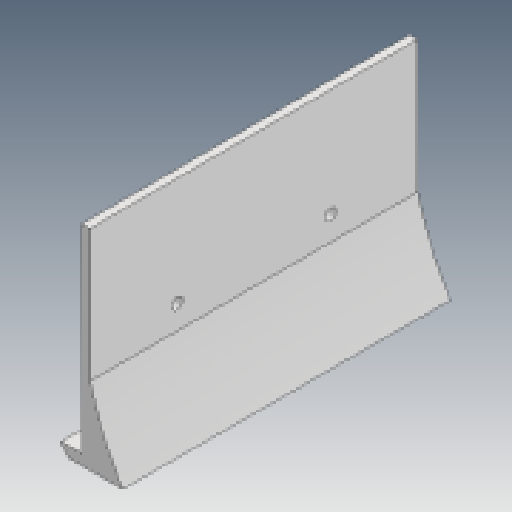
# Autodesk Inventor part: Rampa
Saved by Autodesk Inventor 2026.1 (Build 301233020, 233B)
## iProperties
Created: 2025-11-13
Part Number: Rampa
Material: Genérico
Document SubType Name: Modeling
Designer: Emmanuel Ribeiro
Density: 1 g/cm^3
Appearance: Padrão
Author: Emmanuel Ribeiro
Autodesk Inventor part; units mm, degrees
ref_plane "YZ Plane" through (0, 0, 0) normal (1, 0, 0) x (0, 1, 0)
ref_plane "XZ Plane" through (0, 0, 0) normal (0, 1, 0) x (-1, 0, 0)
ref_plane "XY Plane" through (0, 0, 0) normal (0, 0, 1) x (1, 0, 0)
sketch "Esboço1" plane through (0, 0, 0) normal (0, 0, 1) x (1, 0, 0)
  line L0 (0, 0) -> (10, 0)
  line L1 (0, 51.1555) -> (0, 0)
  line L2 (2, 35) -> (2, 18.8445)
  line L3 (2, 35) -> (2, 51.1555)
  arc A0 (2, 18.8445) -> (10, 0) centre (66.25, 35) ccw
  line L4 (2, 51.1555) -> (0, 51.1555)
  constraints: 10 end point, 2 perpendicular, 2 point on circle, 1 centre point, 1 horizontal
extrude "Extrusão1" add sketch "Esboço1" along normal blind 80
sketch "Esboço2" plane through (0, 0, 80) normal (0, 0, 1) x (1, 0, 0)
  line L0 (0, 0) -> (10, 0) projected
  line L1 (0, 0) -> (-3, 0)
  line L2 (-5, 2) -> (-5, 2.6)
  line L3 (-5, 2.6) -> (0, 2.6)
  line L4 (-3, 0) -> (-5, 2)
  line L5 (0, 51.1555) -> (0, 0) projected
  line L6 (0, 2.6) -> (0, 0)
  point P0 (-5, 0)
  dimension "d5" = 5
  dimension "d6" = 2.6
  dimension "d7" = 2
  dimension "d8" = 2
  constraints: 10 end point, 2 perpendicular, 2 point on line, 1 horizontal, 1 vertical
  measures "d5" distance of L0.start point (-5, 0)
  measures "d6" distance of point (-5, 0) L2.end
  measures "d7" distance of L1.end point (-5, 0)
  measures "d8" distance of L2.start point (-5, 0)
extrude "Extrusão2" add sketch "Esboço2" against normal blind 80
sketch "Esboço3" plane through (2, 18.8445, 0) normal (1, 0, 0) x (0, 0, -1)
  line L0 (0, 0) -> (-80, 0) projected
  line L1 (-2.5, 11.7555) -> (-77.5, 11.7555) projected
  line L2 (-2.5, 11.7555) -> (-2.5, -13.7445) projected
  line L3 (-77.5, -13.7445) -> (-2.5, -13.7445) projected
  line L4 (-77.5, 11.7555) -> (-77.5, -13.7445) projected
  line L5 (-77.5, 11.7555) -> (-40, 0) construction
  line L6 (-40, 0) -> (-2.5, 11.7555) construction
  circle A0 centre (-58.75, 5.8777) radius 1.4
  circle A1 centre (-21.25, 5.8777) radius 1.4
  point P0 (0, -18.8445)
  dimension "d11" = 2.8
  dimension "d12" = 2.8
  constraints: 4 end point, 3 midpoint, 2 centre point
  measures "d11" diameter of A0
  measures "d12" diameter of A1
extrude "Extrusão3" cut sketch "Esboço3" against normal blind 80 contours A0 | A1
equation "\"d8\" = d7"
